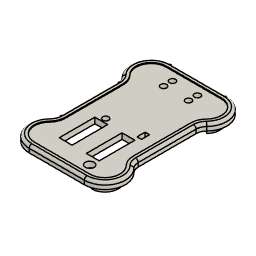
tiny-scarab-v0.3-cover (Autodesk Fusion 360 design; units mm, degrees)
Autodesk Fusion 360 part; units mm, degrees
sketch "drawing" plane through (0, 0, 0) normal (0, 0, 1) x (1, 0, 0)
  circle A0 centre (76.25, -27.495) radius 1.5
  circle A1 centre (114.25, -27.495) radius 1.5
  circle A2 centre (76.25, -87.495) radius 1.5
  circle A3 centre (114.25, -87.495) radius 1.5
  line L0 (79.75, -93.495) -> (110.75, -93.495)
  line L1 (77.25, -41.2424) -> (77.25, -73.7476)
  line L2 (113.25, -41.2424) -> (113.25, -73.7476)
  arc A4 (79.75, -21.495) -> (74.3929, -34.2439) centre (79.75, -28.995) ccw
  arc A5 (116.1071, -34.2439) -> (110.75, -21.495) centre (110.75, -28.995) ccw
  arc A6 (74.3929, -80.7461) -> (79.75, -93.495) centre (79.75, -85.995) ccw
  arc A7 (110.75, -93.495) -> (116.1071, -80.7461) centre (110.75, -85.995) ccw
  circle A8 centre (76.25, -27.495) radius 3
  circle A9 centre (114.25, -27.495) radius 3
  circle A10 centre (76.25, -87.495) radius 3
  circle A11 centre (114.25, -87.495) radius 3
  line L3 (72.25, -21.495) -> (72.25, -93.495) construction
  line L4 (118.25, -21.495) -> (118.25, -93.495) construction
  circle A12 centre (88.25, -25.495) radius 1.7
  circle A13 centre (88.25, -30.495) radius 1.7
  circle A14 centre (83.25, -26.495) radius 1.5
  circle A15 centre (83.25, -34.995) radius 1.5
  line L5 (95.25, -21.495) -> (95.25, -93.495) construction
  circle A16 centre (106.68, -60.325) radius 0.25 construction
  line L6 (104.93, -55.8) -> (108.43, -55.8) construction
  line L7 (108.43, -55.8) -> (108.43, -64.85) construction
  line L8 (108.43, -64.85) -> (104.93, -64.85) construction
  line L9 (104.93, -64.85) -> (104.93, -55.8) construction
  arc A17 (77.25, -41.2424) -> (74.3929, -34.2439) centre (67.25, -41.2424) ccw
  line L10 (79.75, -28.995) -> (79.75, -21.495) construction
  line L11 (79.75, -28.995) -> (74.3929, -34.2439) construction
  line L12 (67.25, -41.2424) -> (77.25, -41.2424) construction
  line L13 (67.25, -41.2424) -> (74.3929, -34.2439) construction
  arc A18 (116.1071, -34.2439) -> (113.25, -41.2424) centre (123.25, -41.2424) ccw
  arc A19 (74.3929, -80.7461) -> (77.25, -73.7476) centre (67.25, -73.7476) ccw
  arc A20 (113.25, -73.7476) -> (116.1071, -80.7461) centre (123.25, -73.7476) ccw
  circle A21 centre (102.25, -25.495) radius 1.7
  circle A22 centre (102.25, -30.495) radius 1.7
  circle A23 centre (87.75, -62.495) radius 1.7
  line L14 (105.43, -58.075) -> (107.93, -58.075)
  line L15 (107.93, -58.075) -> (107.93, -62.575)
  line L16 (107.93, -62.575) -> (105.43, -62.575)
  line L17 (105.43, -62.575) -> (105.43, -58.075)
  line L18 (105.93, -60.575) -> (107.43, -60.575) construction
  line L19 (107.43, -60.575) -> (107.43, -62.075) construction
  line L20 (107.43, -62.075) -> (105.93, -62.075) construction
  line L21 (105.93, -62.075) -> (105.93, -60.575) construction
  line L22 (105.93, -58.575) -> (107.43, -58.575) construction
  line L23 (107.43, -58.575) -> (107.43, -60.075) construction
  line L24 (107.43, -60.075) -> (105.93, -60.075) construction
  line L25 (105.93, -60.075) -> (105.93, -58.575) construction
  line L26 (106.68, -60.075) -> (106.68, -60.575) construction
  line L27 (81, -24.245) -> (85.5, -24.245) construction
  line L28 (85.5, -24.245) -> (85.5, -28.745) construction
  line L29 (85.5, -28.745) -> (81, -28.745) construction
  line L30 (81, -28.745) -> (81, -24.245) construction
  circle A24 centre (88.25, -25.495) radius 1.9 construction
  circle A25 centre (88.25, -30.495) radius 1.9 construction
  circle A26 centre (102.25, -25.495) radius 1.9 construction
  circle A27 centre (102.25, -30.495) radius 1.9 construction
  circle A28 centre (87.75, -62.495) radius 1.9 construction
  line L31 (81, -32.745) -> (85.5, -32.745) construction
  line L32 (85.5, -32.745) -> (85.5, -37.245) construction
  line L33 (85.5, -37.245) -> (81, -37.245) construction
  line L34 (81, -37.245) -> (81, -32.745) construction
  circle A29 centre (107.25, -26.495) radius 1.5
  line L35 (105, -24.245) -> (109.5, -24.245) construction
  line L36 (109.5, -24.245) -> (109.5, -28.745) construction
  line L37 (109.5, -28.745) -> (105, -28.745) construction
  line L38 (105, -28.745) -> (105, -24.245) construction
  circle A30 centre (105.75, -89.495) radius 1.5
  line L39 (103.5, -87.245) -> (108, -87.245) construction
  line L40 (108, -87.245) -> (108, -91.745) construction
  line L41 (108, -91.745) -> (103.5, -91.745) construction
  line L42 (103.5, -91.745) -> (103.5, -87.245) construction
  line L43 (85.03, -65.882) -> (90.23, -65.882) construction
  line L44 (90.23, -65.882) -> (90.23, -83.882) construction
  line L45 (90.23, -83.882) -> (85.03, -83.882) construction
  line L46 (85.03, -83.882) -> (85.03, -65.882) construction
  line L47 (100.27, -65.882) -> (105.47, -65.882) construction
  line L48 (105.47, -65.882) -> (105.47, -83.882) construction
  line L49 (105.47, -83.882) -> (100.27, -83.882) construction
  line L50 (100.27, -83.882) -> (100.27, -65.882) construction
  line L51 (91.23, -64.882) -> (91.23, -84.882)
  line L52 (91.23, -84.882) -> (84.03, -84.882)
  line L53 (84.03, -84.882) -> (84.03, -64.882)
  line L54 (84.03, -64.882) -> (91.23, -64.882)
  line L55 (106.47, -84.882) -> (99.27, -84.882)
  line L56 (99.27, -84.882) -> (99.27, -64.882)
  line L57 (99.27, -64.882) -> (106.47, -64.882)
  line L58 (106.47, -64.882) -> (106.47, -84.882)
  line L59 (89.25, -21.495) -> (89.25, -18.495)
  line L60 (101.25, -21.495) -> (101.25, -18.495)
  line L61 (90.25, -17.495) -> (100.25, -17.495)
  line L62 (79.75, -21.495) -> (89.25, -21.495)
  line L63 (101.25, -21.495) -> (110.75, -21.495)
  line L64 (89.25, -21.495) -> (101.25, -21.495) construction
  line L65 (110.75, -21.495) -> (110.75, -28.995) construction
  arc A31 (90.25, -17.495) -> (89.25, -18.495) centre (90.25, -18.495) ccw
  arc A32 (101.25, -18.495) -> (100.25, -17.495) centre (100.25, -18.495) ccw
  line L66 (98.975, -19.674) -> (98.975, -20.274) construction
  arc A33 (98.975, -20.274) -> (100.175, -20.274) centre (99.575, -20.274) ccw construction
  line L67 (100.175, -20.274) -> (100.175, -19.674) construction
  arc A34 (100.175, -19.674) -> (98.975, -19.674) centre (99.575, -19.674) ccw construction
  line L68 (99.575, -19.674) -> (99.575, -20.274) construction
  line L69 (99.575, -19.074) -> (99.575, -20.874) construction
  line L70 (99.975, -20.274) -> (99.975, -19.674)
  arc A35 (99.975, -19.674) -> (99.175, -19.674) centre (99.575, -19.674) ccw
  line L71 (99.175, -19.674) -> (99.175, -20.274)
  arc A36 (99.175, -20.274) -> (99.975, -20.274) centre (99.575, -20.274) ccw
  line L72 (99.575, -20.274) -> (99.575, -19.674) construction
  line L73 (91.525, -20.274) -> (91.525, -19.674) construction
  arc A37 (91.525, -19.674) -> (90.325, -19.674) centre (90.925, -19.674) ccw construction
  line L74 (90.325, -19.674) -> (90.325, -20.274) construction
  arc A38 (90.325, -20.274) -> (91.525, -20.274) centre (90.925, -20.274) ccw construction
  line L75 (90.925, -20.274) -> (90.925, -19.674) construction
  line L76 (91.325, -20.274) -> (91.325, -19.674)
  arc A39 (91.325, -19.674) -> (90.525, -19.674) centre (90.925, -19.674) ccw
  line L77 (90.525, -19.674) -> (90.525, -20.274)
  arc A40 (90.525, -20.274) -> (91.325, -20.274) centre (90.925, -20.274) ccw
  line L78 (90.925, -20.274) -> (90.925, -19.674) construction
  line L79 (90.925, -19.074) -> (90.925, -20.874) construction
  line L80 (90.925, -19.274) -> (99.575, -19.274) construction
  line L81 (90.925, -20.674) -> (99.575, -20.674) construction
  line L82 (90.925, -19.074) -> (99.575, -19.074) construction
  line L83 (90.925, -20.874) -> (99.575, -20.874) construction
  line L84 (99.975, -24.574) -> (99.975, -23.774)
  arc A41 (99.975, -23.774) -> (99.175, -23.774) centre (99.575, -23.774) ccw
  line L85 (99.175, -23.774) -> (99.175, -24.574)
  arc A42 (99.175, -24.574) -> (99.975, -24.574) centre (99.575, -24.574) ccw
  line L86 (99.575, -24.574) -> (99.575, -23.774) construction
  line L87 (99.575, -23.374) -> (99.575, -24.974) construction
  line L88 (91.325, -24.574) -> (91.325, -23.774)
  arc A43 (91.325, -23.774) -> (90.525, -23.774) centre (90.925, -23.774) ccw
  line L89 (90.525, -23.774) -> (90.525, -24.574)
  arc A44 (90.525, -24.574) -> (91.325, -24.574) centre (90.925, -24.574) ccw
  line L90 (90.925, -24.574) -> (90.925, -23.774) construction
  line L91 (90.925, -23.374) -> (90.925, -24.974) construction
  line L92 (90.925, -19.974) -> (90.925, -24.174) construction
  line L93 (99.575, -19.974) -> (99.575, -24.174) construction
  line L94 (91.525, -24.574) -> (91.525, -23.774) construction
  arc A45 (91.525, -23.774) -> (90.325, -23.774) centre (90.925, -23.774) ccw construction
  line L95 (90.325, -23.774) -> (90.325, -24.574) construction
  arc A46 (90.325, -24.574) -> (91.525, -24.574) centre (90.925, -24.574) ccw construction
  line L96 (90.925, -24.574) -> (90.925, -23.774) construction
  line L97 (100.175, -24.574) -> (100.175, -23.774) construction
  arc A47 (100.175, -23.774) -> (98.975, -23.774) centre (99.575, -23.774) ccw construction
  line L98 (98.975, -23.774) -> (98.975, -24.574) construction
  arc A48 (98.975, -24.574) -> (100.175, -24.574) centre (99.575, -24.574) ccw construction
  line L99 (99.575, -24.574) -> (99.575, -23.774) construction
  line L100 (90.925, -23.174) -> (99.575, -23.174) construction
  line L101 (90.925, -25.174) -> (99.575, -25.174) construction
  line L102 (90.925, -23.374) -> (99.575, -23.374) construction
  line L103 (90.925, -24.974) -> (99.575, -24.974) construction
  line L104 (90.75, -17.495) -> (99.75, -17.495)
  line L105 (99.75, -17.495) -> (99.75, -24.845)
  line L106 (99.75, -24.845) -> (90.75, -24.845)
  line L107 (90.75, -24.845) -> (90.75, -17.495)
  point P0 (87.63, -74.882)
  point P1 (102.87, -74.882)
  point P2 (99.575, -19.974)
  point P3 (99.575, -19.974)
  point P4 (90.925, -19.974)
  point P5 (90.925, -19.974)
  point P6 (99.575, -24.174)
  point P7 (90.925, -24.174)
  point P8 (90.925, -24.174)
  point P9 (99.575, -24.174)
  dimension "d1" = 76.25
  dimension "d2" = 3
  dimension "d3" = 27.495
  dimension "d4" = 3
  dimension "d5" = 38
  dimension "d6" = 27.495
  dimension "d7" = 1.5
  dimension "d8" = 3.5
  dimension "d9" = 15
  dimension "d10" = 3.5
  dimension "d11" = 1.5
  dimension "d12" = 15
  dimension "d13" = 60
  dimension "d14" = 3
  dimension "d15" = 76.25
  dimension "d16" = 38
  dimension "d17" = 60
  dimension "d18" = 3
  dimension "d19" = 3.5
  dimension "d20" = 1.5
  dimension "d21" = 3.5
  dimension "d22" = 1.5
  dimension "d23" = 15
  dimension "d24" = 15
  dimension "d31" = 6
  dimension "d32" = 6
  dimension "d33" = 6
  dimension "d34" = 6
  dimension "d35" = 72
  dimension "d36" = 46
  dimension "d37" = 6
  dimension "d38" = 5
  dimension "d39" = 5
  dimension "d40" = 4
  dimension "d41" = 4
  dimension "d42" = 12
  dimension "d43" = 2
  dimension "d44" = 3.4
  dimension "d45" = 5
  dimension "d46" = 3.4
  dimension "d47" = 7
  dimension "d48" = 1
  dimension "d49" = 3
  dimension "d50" = 3
  dimension "d51" = 8.5
  dimension "d52" = 19
  dimension "d56" = 106.68
  dimension "d57" = 60.325
  dimension "d58" = 0.5
  dimension "d59" = 4.525
  dimension "d62" = 1.75
  dimension "d75" = 20
  dimension "d76" = 134.415
  dimension "d77" = 44.415
  dimension "d78" = 20
  dimension "d79" = 20
  dimension "d80" = 20
  dimension "d92" = 3.4
  dimension "d93" = 3.4
  dimension "d94" = 14
  dimension "d95" = 3.4
  dimension "d96" = 32
  dimension "d97" = 0.5
  dimension "d98" = 1.25
  dimension "d100" = 1.5
  dimension "d101" = 0.75
  dimension "d102" = 1.5
  dimension "d103" = 0.75
  dimension "d104" = 3.5
  dimension "d105" = 0.5
  dimension "d106" = 1.5
  dimension "d107" = 3.5
  dimension "d108" = 9.05
  dimension "d109" = 2.25
  dimension "d110" = 2.25
  dimension "d111" = 2.5
  dimension "d112" = 0.5
  dimension "d113" = 0.5
  dimension "d114" = 2.25
  dimension "d115" = 4.5
  dimension "d116" = 4.5
  dimension "d117" = 2.25
  dimension "d118" = 3.8
  dimension "d119" = 3.8
  dimension "d120" = 3.8
  dimension "d121" = 3.8
  dimension "d122" = 3.8
  dimension "d123" = 4.5
  dimension "d124" = 4.5
  dimension "d125" = 2.25
  dimension "d126" = 2.25
  dimension "d127" = 5
  dimension "d128" = 3
  dimension "d129" = 2.25
  dimension "d130" = 2.25
  dimension "d131" = 4.5
  dimension "d132" = 4.5
  dimension "d133" = 105.75
  dimension "d134" = 89.495
  dimension "d135" = 3
  dimension "d136" = 4.5
  dimension "d137" = 4.5
  dimension "d138" = 2.25
  dimension "d139" = 2.25
  dimension "d140" = 4
  dimension "d141" = 12.5
  dimension "d142" = 18
  dimension "d143" = 18
  dimension "d144" = 5.2
  dimension "d145" = 5.2
  dimension "d146" = 102.87
  dimension "d147" = 87.63
  dimension "d148" = 74.882
  dimension "d149" = 2.6
  dimension "d150" = 2.6
  dimension "d151" = 9
  dimension "d152" = 9
  dimension "d153" = -1
  dimension "d154" = -1
  dimension "d200" = 18
  dimension "d201" = 18
  dimension "d202" = 12
  dimension "d203" = 6
  dimension "d204" = 4
  dimension "d205" = 1
  dimension "d206" = 1
  dimension "d207" = 1.675
  dimension "d208" = 2.479
  dimension "d209" = 1.2
  dimension "d210" = 1.8
  dimension "d211" = 0.8
  dimension "d212" = 1.2
  dimension "d213" = 2.479
  dimension "d214" = 1.675
  dimension "d215" = 0.4
  dimension "d216" = 0.8
  dimension "d217" = 1.8
  dimension "d218" = 1.2
  dimension "d219" = 1.2
  dimension "d220" = 1.579
  dimension "d226" = 1.8
  dimension "d227" = 1.4
  dimension "d236" = 1.6
  dimension "d237" = 0.8
  dimension "d238" = 1.6
  dimension "d239" = 0.8
  dimension "d240" = 4.2
  dimension "d241" = 4.2
  dimension "d242" = 1.2
  dimension "d243" = 1.2
  dimension "d245" = 1.6
  dimension "d246" = 2
  dimension "d247" = 4.5
  dimension "d248" = 4.5
  dimension "d249" = 7.35
  constraint tangent A4 L62
  constraint tangent A5 L62
  constraint tangent L0 A6
  constraint tangent L0 A7
  constraint concentric A0 A8
  constraint concentric A1 A9
  constraint concentric A2 A10
  constraint concentric A3 A11
  constraint vertical L3
  constraint tangent A6 L3
  constraint coincident L3.start L62
  constraint coincident L0 L3.end
  constraint vertical L4
  constraint coincident L4.start L62
  constraint coincident L0 L4.end
  constraint tangent A7 L4
  constraint vertical A12.centre A13.centre
  constraint vertical A14.centre A15.centre
  constraint coincident L5.start L62
  constraint coincident L0 L5.end
  constraint perpendicular L0 L5
  constraint horizontal L6
  constraint vertical L7
  constraint horizontal L8
  constraint vertical L9
  constraint tangent A4 A17
  constraint tangent L1 A17
  constraint coincident A4.centre L10.start
  constraint coincident A17.centre L12.start
  constraint tangent A5 A18
  constraint tangent L2 A18
  constraint tangent A6 A19
  constraint tangent L1 A19
  constraint tangent A7 A20
  constraint tangent L2 A20
  constraint vertical A21.centre A22.centre
  constraint horizontal A12.centre A21.centre
  constraint horizontal A13.centre A22.centre
  constraint horizontal L14
  constraint vertical L15
  constraint horizontal L16
  constraint vertical L17
  constraint horizontal L18
  constraint vertical L19
  constraint horizontal L20
  constraint vertical L21
  constraint horizontal L22
  constraint vertical L23
  constraint horizontal L24
  constraint vertical L25
  constraint midpoint L24 L26.start
  constraint midpoint L18 L26.end
  constraint midpoint A16.centre L26
  constraint horizontal L27
  constraint vertical L28
  constraint horizontal L29
  constraint vertical L30
  constraint concentric A12 A24
  constraint concentric A13 A25
  constraint concentric A21 A26
  constraint concentric A22 A27
  constraint concentric A23 A28
  constraint horizontal L31
  constraint vertical L32
  constraint horizontal L33
  constraint vertical L34
  constraint horizontal A14.centre A29.centre
  constraint horizontal L35
  constraint vertical L36
  constraint horizontal L37
  constraint vertical L38
  constraint horizontal L39
  constraint vertical L40
  constraint horizontal L41
  constraint vertical L42
  constraint horizontal L43
  constraint vertical L44
  constraint horizontal L45
  constraint vertical L46
  constraint horizontal L47
  constraint vertical L48
  constraint horizontal L49
  constraint vertical L50
  constraint horizontal P0 P1
  constraint vertical L60
  constraint vertical L59
  constraint horizontal L61
  constraint perpendicular L60 L64
  constraint coincident A5.centre L65.end
  constraint perpendicular L63 L65
  constraint tangent L59 A31
  constraint tangent L61 A31
  constraint tangent L60 A32
  constraint tangent L61 A32
  constraint tangent L66 A33
  constraint tangent A33 L67
  constraint parallel L66 L67
  constraint tangent L67 A34
  constraint tangent L66 A34
  constraint vertical L68
  constraint midpoint L68 P3
  constraint midpoint A34 L69.start
  constraint midpoint A33 L69.end
  constraint tangent L70 A35
  constraint tangent A35 L71
  constraint parallel L70 L71
  constraint tangent L71 A36
  constraint tangent L70 A36
  constraint coincident A34.centre L68.start
  constraint parallel L69 L72
  constraint coincident P3 P2
  constraint tangent L73 A37
  constraint tangent A37 L74
  constraint parallel L73 L74
  constraint tangent L74 A38
  constraint tangent L73 A38
  constraint vertical L75
  constraint midpoint L75 P5
  constraint collinear L66.end L70.start L71.end
  constraint collinear L66.end A33.end L70.start
  constraint tangent L76 A39
  constraint tangent A39 L77
  constraint parallel L76 L77
  constraint tangent L77 A40
  constraint tangent L76 A40
  constraint coincident A37.centre L75.end
  constraint parallel L75 L78
  constraint coincident P5 P4
  constraint midpoint L78 P5
  constraint midpoint A37 L79.start
  constraint midpoint A38 L79.end
  constraint midpoint A39 L80.start
  constraint midpoint A35 L80.end
  constraint midpoint A40 L81.start
  constraint midpoint A36 L81.end
  constraint tangent L84 A41
  constraint tangent A41 L85
  constraint parallel L84 L85
  constraint tangent L85 A42
  constraint tangent L84 A42
  constraint parallel L79 L86
  constraint midpoint L86 P9
  constraint midpoint A41 L87.start
  constraint midpoint A42 L87.end
  constraint tangent L88 A43
  constraint tangent A43 L89
  constraint parallel L88 L89
  constraint tangent L89 A44
  constraint tangent L88 A44
  constraint perpendicular L64 L90
  constraint midpoint L90 P8
  constraint midpoint A43 L91.start
  constraint midpoint A44 L91.end
  constraint coincident P8 P7
  constraint vertical L92
  constraint coincident P9 P6
  constraint vertical L93
  constraint tangent L94 A45
  constraint tangent A45 L95
  constraint parallel L94 L95
  constraint tangent L95 A46
  constraint tangent L94 A46
  constraint coincident L92 A43.centre
  constraint parallel L92 L96
  constraint midpoint L96 P8
  constraint coincident A43.centre L90.end
  constraint tangent L97 A47
  constraint tangent A47 L98
  constraint parallel L97 L98
  constraint tangent L98 A48
  constraint tangent L97 A48
  constraint coincident L93 A41.centre
  constraint parallel L93 L99
  constraint midpoint L99 P9
  constraint coincident A41.centre L86.end
  constraint midpoint A45 L100.start
  constraint midpoint A47 L100.end
  constraint midpoint A46 L101.start
  constraint midpoint A48 L101.end
  constraint horizontal L104
  constraint vertical L105
  constraint horizontal L106
  constraint vertical L107
  constraint collinear L61 L104
  measures "d1" horizontal distance of origin A0.centre
  measures "d2" diameter of A0
  measures "d3" vertical distance of origin A0.centre
  measures "d4" diameter of A1
  measures "d5" horizontal distance of A0.centre A1.centre
  measures "d6" vertical distance of origin A1.centre
  measures "d7" vertical distance of A0.centre A4.centre
  measures "d8" horizontal distance of A0.centre A4.centre
  measures "d9" diameter of A4
  measures "d10" horizontal distance of A1.centre A5.centre
  measures "d11" vertical distance of A1.centre A5.centre
  measures "d12" diameter of A5
  measures "d13" vertical distance of A0.centre A2.centre
  measures "d14" diameter of A2
  measures "d15" horizontal distance of origin A2.centre
  measures "d16" horizontal distance of A2.centre A3.centre
  measures "d17" distance of A1.centre A3.centre
  measures "d18" diameter of A3
  measures "d19" horizontal distance of A3.centre A7.centre
  measures "d20" vertical distance of A3.centre A7.centre
  measures "d21" horizontal distance of A2.centre A6.centre
  measures "d22" vertical distance of A2.centre A6.centre
  measures "d23" diameter of A6
  measures "d24" diameter of A7
  measures "d31" diameter of A8
  measures "d32" diameter of A9
  measures "d33" diameter of A10
  measures "d34" diameter of A11
  measures "d35" distance of L0 L62
  measures "d36" distance of L3 L4
  measures "d37" distance of A1.centre L62
  measures "d38" distance of L2 L4
  measures "d39" distance of L1 L3
  measures "d40" distance of A2.centre L3
  measures "d41" distance of A3.centre L4
  measures "d42" horizontal distance of A0.centre A12.centre
  measures "d43" vertical distance of A0.centre A12.centre
  measures "d44" diameter of A12
  measures "d45" vertical distance of A12.centre A13.centre
  measures "d46" diameter of A13
  measures "d47" horizontal distance of A0.centre A14.centre
  measures "d48" vertical distance of A0.centre A14.centre
  measures "d49" diameter of A14
  measures "d50" diameter of A15
  measures "d51" distance of A14.centre A15.centre
  measures "d52" distance of A2.centre L5
  measures "d56" horizontal distance of origin A16.centre
  measures "d57" vertical distance of origin A16.centre
  measures "d58" diameter of A16
  measures "d59" distance of A16.centre L6
  measures "d62" distance of A16.centre L7
  measures "d75" diameter of A17
  measures "d76" angle of L10 L11
  measures "d77" angle of L12 L13
  measures "d78" diameter of A18
  measures "d79" diameter of A19
  measures "d80" diameter of A20
  measures "d92" diameter of A21
  measures "d93" diameter of A22
  measures "d94" horizontal distance of A12.centre A21.centre
  measures "d95" diameter of A23
  measures "d96" vertical distance of A13.centre A23.centre
  measures "d97" horizontal distance of A13.centre A23.centre
  measures "d98" distance of A16.centre L15
  measures "d100" distance of L19 L21
  measures "d101" distance of A16.centre L19
  measures "d102" distance of L23 L25
  measures "d103" distance of A16.centre L23
  measures "d104" distance of L20 L22
  measures "d105" distance of L18 L24
  measures "d106" distance of L18 L20
  measures "d107" distance of L7 L9
  measures "d108" distance of L6 L8
  measures "d109" distance of A16.centre L14
  measures "d110" distance of A16.centre L16
  measures "d111" distance of L15 L17
  measures "d112" distance of L17 L25
  measures "d113" distance of L16 L20
  measures "d114" distance of A14.centre L27
  measures "d115" distance of L27 L29
  measures "d116" distance of L28 L30
  measures "d117" distance of A14.centre L30
  measures "d118" diameter of A24
  measures "d119" diameter of A25
  measures "d120" diameter of A26
  measures "d121" diameter of A27
  measures "d122" diameter of A28
  measures "d123" distance of L32 L34
  measures "d124" distance of L31 L33
  measures "d125" distance of A15.centre L32
  measures "d126" distance of A15.centre L33
  measures "d127" horizontal distance of A21.centre A29.centre
  measures "d128" diameter of A29
  measures "d129" distance of A29.centre L35
  measures "d130" distance of A29.centre L36
  measures "d131" distance of L35 L37
  measures "d132" distance of L36 L38
  measures "d133" horizontal distance of origin A30.centre
  measures "d134" vertical distance of origin A30.centre
  measures "d135" diameter of A30
  measures "d136" distance of L40 L42
  measures "d137" distance of L39 L41
  measures "d138" distance of A30.centre L39
  measures "d139" distance of A30.centre L40
  measures "d140" distance of L0 A30.centre
  measures "d141" distance of L4 A30.centre
  measures "d142" distance of L47 L49
  measures "d143" distance of L43 L45
  measures "d144" distance of L44 L46
  measures "d145" distance of L48 L50
  measures "d146" horizontal distance of origin P1
  measures "d147" horizontal distance of origin P0
  measures "d148" vertical distance of origin P0
  measures "d149" distance of L48 P1
  measures "d150" distance of L44 P0
  measures "d151" distance of L47 P1
  measures "d152" distance of L43 P0
  measures "d200" distance of L2 L5
  measures "d201" distance of L1 L5
  measures "d202" distance of L59 L60
  measures "d203" distance of L5 L59
  measures "d204" distance of L61 L62
  measures "d205" radius of A31
  measures "d206" radius of A32
  measures "d207" distance of L60 P3
  measures "d208" distance of L61 P3
  measures "d209" distance of L66 L67
  measures "d210" distance of L69.start L69.end
  measures "d211" diameter of A35
  measures "d212" diameter of A37
  measures "d213" distance of L61 P5
  measures "d214" distance of L59 P5
  measures "d215" radius of A36
  measures "d216" diameter of A39
  measures "d217" distance of L79.start L79.end
  measures "d218" distance of L73 L74
  measures "d219" distance of L66 L67
  measures "d220" distance of L61 L69.start
  measures "d226" distance of L82 L83
  measures "d227" distance of L80 L81
  measures "d236" distance of L87.start L87.end
  measures "d237" distance of L84 L85
  measures "d238" distance of L91.start L91.end
  measures "d239" distance of L88 L89
  measures "d240" vertical distance of P3 P9
  measures "d241" vertical distance of P5 P8
  measures "d242" distance of L97 L98
  measures "d243" distance of L94 L95
  measures "d245" distance of L102 L103
  measures "d246" distance of L100 L101
  measures "d247" distance of L5 L107
  measures "d248" distance of L5 L105
  measures "d249" distance of L104 L106
sketch "board_cutout" plane through (0, 0, 0) normal (0, 0, 1) x (1, 0, 0)
  circle A0 centre (76.25, -27.495) radius 1.5
  circle A1 centre (114.25, -27.495) radius 1.5
  circle A2 centre (76.25, -87.495) radius 1.5
  circle A3 centre (114.25, -87.495) radius 1.5
  arc A4 (79.75, -21.495) -> (74.3929, -34.2439) centre (79.75, -28.995) ccw
  arc A5 (77.25, -41.2424) -> (74.3929, -34.2439) centre (67.25, -41.2424) ccw
  line L0 (77.25, -41.2424) -> (77.25, -73.7476)
  arc A6 (74.3929, -80.7461) -> (77.25, -73.7476) centre (67.25, -73.7476) ccw
  arc A7 (74.3929, -80.7461) -> (79.75, -93.495) centre (79.75, -85.995) ccw
  line L1 (79.75, -93.495) -> (110.75, -93.495)
  arc A8 (110.75, -93.495) -> (116.1071, -80.7461) centre (110.75, -85.995) ccw
  arc A9 (113.25, -73.7476) -> (116.1071, -80.7461) centre (123.25, -73.7476) ccw
  line L2 (113.25, -41.2424) -> (113.25, -73.7476)
  arc A10 (116.1071, -34.2439) -> (113.25, -41.2424) centre (123.25, -41.2424) ccw
  arc A11 (116.1071, -34.2439) -> (110.75, -21.495) centre (110.75, -28.995) ccw
  line L3 (79.75, -21.495) -> (89.25, -21.495)
sketch "board_cutout_4mm_offset" plane through (0, 0, 0) normal (0, 0, 1) x (1, 0, 0)
  arc A0 (79.75, -21.495) -> (74.3929, -34.2439) centre (79.75, -28.995) ccw construction
  arc A1 (77.25, -41.2424) -> (74.3929, -34.2439) centre (67.25, -41.2424) ccw construction
  line L0 (77.25, -41.2424) -> (77.25, -73.7476) construction
  arc A2 (74.3929, -80.7461) -> (77.25, -73.7476) centre (67.25, -73.7476) ccw construction
  arc A3 (74.3929, -80.7461) -> (79.75, -93.495) centre (79.75, -85.995) ccw construction
  line L1 (79.75, -93.495) -> (110.75, -93.495) construction
  arc A4 (110.75, -93.495) -> (116.1071, -80.7461) centre (110.75, -85.995) ccw construction
  arc A5 (113.25, -73.7476) -> (116.1071, -80.7461) centre (123.25, -73.7476) ccw construction
  line L2 (113.25, -41.2424) -> (113.25, -73.7476) construction
  arc A6 (116.1071, -34.2439) -> (113.25, -41.2424) centre (123.25, -41.2424) ccw construction
  arc A7 (116.1071, -34.2439) -> (110.75, -21.495) centre (110.75, -28.995) ccw construction
  arc A8 (117.25, -73.7476) -> (118.9643, -77.9467) centre (123.25, -73.7476) ccw
  arc A9 (110.75, -97.495) -> (118.9643, -77.9467) centre (110.75, -85.995) ccw
  line L3 (79.75, -97.495) -> (110.75, -97.495)
  arc A10 (71.5357, -77.9467) -> (79.75, -97.495) centre (79.75, -85.995) ccw
  arc A11 (71.5357, -77.9467) -> (73.25, -73.7476) centre (67.25, -73.7476) ccw
  line L4 (73.25, -41.2424) -> (73.25, -73.7476)
  arc A12 (73.25, -41.2424) -> (71.5357, -37.0433) centre (67.25, -41.2424) ccw
  arc A13 (79.75, -17.495) -> (71.5357, -37.0433) centre (79.75, -28.995) ccw
  line L5 (79.75, -17.495) -> (110.75, -17.495)
  arc A14 (118.9643, -37.0433) -> (110.75, -17.495) centre (110.75, -28.995) ccw
  arc A15 (118.9643, -37.0433) -> (117.25, -41.2424) centre (123.25, -41.2424) ccw
  line L6 (117.25, -41.2424) -> (117.25, -73.7476)
  line L7 (79.75, -21.495) -> (89.25, -21.495)
  dimension "d183" = 80
  constraint concentric A5 A8
  constraint concentric A4 A9
  constraint concentric A3 A10
  constraint concentric A2 A11
  constraint concentric A1 A12
  constraint concentric A0 A13
  constraint concentric A7 A14
  constraint concentric A6 A15
  constraint tangent A8 L6
  constraint tangent A8 A9
  constraint tangent A10 A11
  constraint tangent A12 A13
  constraint tangent A13 L5
  constraint tangent L5 A14
  constraint tangent A14 A15
  constraint tangent A15 L6
  measures "d183" distance of L3 L5
sketch "pillars" plane through (0, 0, 0) normal (0, 0, 1) x (1, 0, 0)
  arc A0 (79.75, -21.495) -> (74.3929, -34.2439) centre (79.75, -28.995) ccw
  arc A1 (77.25, -41.2424) -> (74.3929, -34.2439) centre (67.25, -41.2424) ccw construction
  line L0 (77.25, -41.2424) -> (77.25, -73.7476) construction
  arc A2 (74.3929, -80.7461) -> (77.25, -73.7476) centre (67.25, -73.7476) ccw construction
  arc A3 (74.3929, -80.7461) -> (79.75, -93.495) centre (79.75, -85.995) ccw
  line L1 (79.75, -93.495) -> (110.75, -93.495) construction
  arc A4 (110.75, -93.495) -> (116.1071, -80.7461) centre (110.75, -85.995) ccw
  arc A5 (113.25, -73.7476) -> (116.1071, -80.7461) centre (123.25, -73.7476) ccw construction
  line L2 (113.25, -41.2424) -> (113.25, -73.7476) construction
  arc A6 (116.1071, -34.2439) -> (113.25, -41.2424) centre (123.25, -41.2424) ccw construction
  arc A7 (116.1071, -34.2439) -> (110.75, -21.495) centre (110.75, -28.995) ccw
  circle A8 centre (76.25, -27.495) radius 1.5 construction
  circle A9 centre (114.25, -27.495) radius 1.5 construction
  circle A10 centre (76.25, -27.495) radius 3 construction
  circle A11 centre (114.25, -27.495) radius 3 construction
  circle A12 centre (76.25, -87.495) radius 1.5 construction
  circle A13 centre (76.25, -87.495) radius 3 construction
  circle A14 centre (114.25, -87.495) radius 1.5 construction
  circle A15 centre (114.25, -87.495) radius 3 construction
  spline S0 degree 2 poles (79.75, -21.495) (79.75, -28.995) (74.3929, -34.2439) knots 0 0 0 1.458918 1.458918 1.458918 weights 1 4 1
  spline S1 degree 2 poles (110.75, -21.495) (110.75, -28.995) (116.1071, -34.2439) knots 0 0 0 1.458918 1.458918 1.458918 weights 1 4 1
  spline S2 degree 2 poles (74.3929, -80.7461) (79.75, -85.995) (79.75, -93.495) knots 0 0 0 1.458918 1.458918 1.458918 weights 1 4 1
  spline S3 degree 2 poles (110.75, -93.495) (110.75, -85.995) (116.1071, -80.7461) knots 0 0 0 1.458918 1.458918 1.458918 weights 1 4 1
  line L3 (79.75, -21.495) -> (89.25, -21.495)
  constraint coincident A0.end A1.end
  constraint coincident A0.start S0.start
  constraint coincident A6.start A7.start
  constraint coincident A7.end S1.start
  constraint coincident A3.end L1.start
  constraint coincident A2.start A3.start
  constraint coincident A4.end A5.end
  constraint coincident L1.end A4.start
sketch "srew_holes" plane through (0, 0, 0) normal (0, 0, 1) x (1, 0, 0)
  circle A0 centre (76.25, -27.495) radius 1.5
  circle A1 centre (114.25, -27.495) radius 1.5
  circle A2 centre (76.25, -87.495) radius 1.5
  circle A3 centre (114.25, -87.495) radius 1.5
  dimension "d250" = 3
  dimension "d251" = 60
  dimension "d252" = 38
  measures "d250" diameter of A0
  measures "d251" distance of A0.centre A2.centre
  measures "d252" distance of A0.centre A1.centre
extrude "Extrude5" add sketch "pillars" along normal blind 4 makes body 1 at (116.0352, -23.6737, 2.6667) makes body 2 at (118.1619, -87.1412, 2.6667) makes body 3 at (72.9424, -32.1424, 2.6667) makes body 4 at (72.403, -87.5019, 2.6667)
extrude "Extrude6" add sketch "board_cutout_4mm_offset" along normal blind 3.7 from surface at 4 separate body makes body 5
sketch "led_cutouts" plane through (0, 0, 0) normal (0, 0, 1) x (1, 0, 0)
  circle A0 centre (88.25, -25.495) radius 1.7
  circle A1 centre (88.25, -30.495) radius 1.7
  circle A2 centre (102.25, -25.495) radius 1.7
  circle A3 centre (102.25, -30.495) radius 1.7
  circle A4 centre (87.75, -62.495) radius 1.7
sketch "button_cutouts" plane through (0, 0, 0) normal (0, 0, 1) x (1, 0, 0)
  circle A0 centre (83.25, -26.495) radius 1.5 construction
  circle A1 centre (83.25, -34.995) radius 1.5 construction
  circle A2 centre (107.25, -26.495) radius 1.5 construction
  circle A3 centre (105.75, -89.495) radius 1.5 construction
  line L0 (105.43, -58.075) -> (107.93, -58.075)
  line L1 (105.43, -62.575) -> (105.43, -58.075)
  line L2 (107.93, -62.575) -> (105.43, -62.575)
  line L3 (107.93, -58.075) -> (107.93, -62.575)
  circle A4 centre (105.75, -89.495) radius 2.5
  dimension "d185" = 3
  dimension "d186" = 1
  dimension "d187" = 5
  measures "d185" diameter of A3
  measures "d187" diameter of A4
sketch "pinheader_cutouts" plane through (0, 0, 0) normal (0, 0, 1) x (1, 0, 0)
  line L0 (91.23, -84.882) -> (84.03, -84.882)
  line L1 (84.03, -84.882) -> (84.03, -64.882)
  line L2 (84.03, -64.882) -> (91.23, -64.882)
  line L3 (91.23, -64.882) -> (91.23, -84.882)
  line L4 (99.27, -64.882) -> (106.47, -64.882)
  line L5 (99.27, -84.882) -> (99.27, -64.882)
  line L6 (106.47, -84.882) -> (99.27, -84.882)
  line L7 (106.47, -64.882) -> (106.47, -84.882)
extrude "Extrude8" cut sketch "led_cutouts" along normal through all bodies 5
extrude "Extrude9" cut sketch "button_cutouts" along normal through all bodies 5
extrude "Extrude10" cut sketch "pinheader_cutouts" along normal through all bodies 5
sketch "screw_sinkholes" plane through (0, 0, 0) normal (0, 0, 1) x (1, 0, 0)
  circle A0 centre (76.25, -27.495) radius 1.5 construction
  circle A1 centre (114.25, -27.495) radius 1.5 construction
  circle A2 centre (76.25, -87.495) radius 1.5 construction
  circle A3 centre (114.25, -87.495) radius 1.5 construction
  circle A4 centre (76.25, -27.495) radius 3
  circle A5 centre (114.25, -27.495) radius 3
  circle A6 centre (76.25, -87.495) radius 3
  circle A7 centre (114.25, -87.495) radius 3
  dimension "d158" = 3
  dimension "d159" = 3
  dimension "d160" = 3
  dimension "d161" = 3
  dimension "d162" = 6
  dimension "d163" = 6
  dimension "d164" = 6
  dimension "d165" = 6
  constraint concentric A0 A4
  constraint concentric A1 A5
  constraint concentric A2 A6
  constraint concentric A3 A7
  measures "d158" diameter of A2
  measures "d159" diameter of A3
  measures "d160" diameter of A0
  measures "d161" diameter of A1
  measures "d162" diameter of A4
  measures "d163" diameter of A5
  measures "d164" diameter of A6
  measures "d165" diameter of A7
sketch "screw_holes_2.26mm" plane through (0, 0, 0) normal (0, 0, 1) x (1, 0, 0)
  circle A0 centre (76.25, -87.495) radius 1.5 construction
  circle A1 centre (114.25, -87.495) radius 1.5 construction
  circle A2 centre (114.25, -27.495) radius 1.5 construction
  circle A3 centre (76.25, -27.495) radius 1.5 construction
  circle A4 centre (76.25, -27.495) radius 1.13
  circle A5 centre (114.25, -27.495) radius 1.13
  circle A6 centre (76.25, -87.495) radius 1.13
  circle A7 centre (114.25, -87.495) radius 1.13
  dimension "d188" = 2.26
  dimension "d189" = 2.26
  dimension "d190" = 2.26
  dimension "d191" = 2.26
  dimension "d253" = 38
  dimension "d254" = 60
  constraint concentric A3 A4
  constraint concentric A2 A5
  constraint concentric A0 A6
  constraint concentric A1 A7
  measures "d188" diameter of A4
  measures "d189" diameter of A5
  measures "d190" diameter of A6
  measures "d191" diameter of A7
  measures "d253" distance of A3.centre A2.centre
  measures "d254" distance of A2.centre A1.centre
extrude "Extrude13" cut sketch "screw_holes_2.26mm" along normal blind 5 bodies 1 2 3 4 5
sketch "membrane_area" plane through (0, 0, 0) normal (0, 0, 1) x (1, 0, 0)
  arc A0 (79.75, -17.495) -> (71.5357, -37.0433) centre (79.75, -28.995) ccw construction
  line L0 (79.75, -17.495) -> (110.75, -17.495) construction
  arc A1 (118.9643, -37.0433) -> (110.75, -17.495) centre (110.75, -28.995) ccw construction
  arc A2 (118.9643, -37.0433) -> (117.25, -41.2424) centre (123.25, -41.2424) ccw construction
  line L1 (117.25, -41.2424) -> (117.25, -73.7476) construction
  arc A3 (117.25, -73.7476) -> (118.9643, -77.9467) centre (123.25, -73.7476) ccw construction
  arc A4 (110.75, -97.495) -> (118.9643, -77.9467) centre (110.75, -85.995) ccw construction
  line L2 (79.75, -97.495) -> (110.75, -97.495) construction
  arc A5 (71.5357, -77.9467) -> (79.75, -97.495) centre (79.75, -85.995) ccw construction
  arc A6 (71.5357, -77.9467) -> (73.25, -73.7476) centre (67.25, -73.7476) ccw construction
  line L3 (73.25, -41.2424) -> (73.25, -73.7476) construction
  arc A7 (73.25, -41.2424) -> (71.5357, -37.0433) centre (67.25, -41.2424) ccw construction
  arc A8 (114.25, -73.7476) -> (116.8214, -80.0462) centre (123.25, -73.7476) ccw
  arc A9 (110.75, -94.495) -> (116.8214, -80.0462) centre (110.75, -85.995) ccw
  line L4 (79.75, -94.495) -> (110.75, -94.495)
  arc A10 (73.6786, -80.0462) -> (79.75, -94.495) centre (79.75, -85.995) ccw
  arc A11 (73.6786, -80.0462) -> (76.25, -73.7476) centre (67.25, -73.7476) ccw
  line L5 (76.25, -41.2424) -> (76.25, -73.7476)
  arc A12 (76.25, -41.2424) -> (73.6786, -34.9438) centre (67.25, -41.2424) ccw
  arc A13 (79.75, -20.495) -> (73.6786, -34.9438) centre (79.75, -28.995) ccw
  line L6 (79.75, -20.495) -> (110.75, -20.495)
  arc A14 (116.8214, -34.9438) -> (110.75, -20.495) centre (110.75, -28.995) ccw
  arc A15 (116.8214, -34.9438) -> (114.25, -41.2424) centre (123.25, -41.2424) ccw
  line L7 (114.25, -41.2424) -> (114.25, -73.7476)
  dimension "d194" = 3
extrude "Extrude14" cut sketch "membrane_area" against normal blind 0.5 from surface at 7.7 bodies 5
fillet "Fillet1" radius 1.5 12 edges at (69.148, -90.45, 7.7) (95.25, -97.495, 7.7) (121.352, -90.45, 7.7) (117.6951, -76.0153, 7.7) (117.25, -57.495, 7.7) (117.6951, -38.9747, 7.7) (121.352, -24.54, 7.7) (95.25, -17.495, 7.7) (69.148, -24.54, 7.7) (72.8049, -38.9747, 7.7) (73.25, -57.495, 7.7) (72.8049, -76.0153, 7.7) on bodies 5
named bodies: "pillar_tr", "pillar_br", "pillar_tl", "pillar_bl", "cover"
